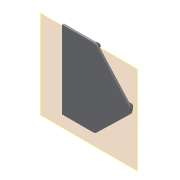
# Autodesk Inventor part: 20_Cube_Insert_VCM_MirrorMount_KES400A_mirror_mount
Saved by Autodesk Inventor 2019.4 (Build 234330000, 330)
## iProperties
Created: 2021-10-15
Part Number: 20_Cube_Insert_VCM_MirrorMount_KES400A_mirror_mount
Material: Generic
Document SubType Name: Modeling
Designer: diederichbenedict
Density: 1 g/cm^3
Appearance: Default
Author: diederichbenedict
Autodesk Inventor part; units mm, degrees
ref_plane "YZ Plane" through (0, 0, 0) normal (1, 0, 0) x (0, 1, 0)
ref_plane "XZ Plane" through (0, 0, 0) normal (0, 1, 0) x (-1, 0, 0)
ref_plane "XY Plane" through (0, 0, 0) normal (0, 0, 1) x (1, 0, 0)
ref_plane "Work Plane1" through (0, 0, -28) normal (0, 0, 1) x (1, 0, 0)
sketch "Sketch1" plane through (0, 0, -28) normal (0, 0, 1) x (1, 0, 0)
  circle A0 centre (27.88, 8) radius 2.6486 projected
  circle A1 centre (27.88, 43) radius 2.6486 projected
  circle A2 centre (44.7, 24.3248) radius 2.6486 projected
  line L0 (27.88, 8) -> (44.7, 24.3248)
  line L1 (44.7, 24.3248) -> (27.88, 43)
  line L2 (27.88, 43) -> (27.88, 8)
  line L3 (46.5446, 22.4242) -> (29.7246, 6.0994)
  line L4 (46.668, 26.0973) -> (29.848, 44.7725)
  line L5 (27.88, 5.3514) -> (11.88, 5.3514)
  line L6 (27.88, 5.3514) -> (43.88, 5.3514) construction
  line L7 (11.88, 5.3514) -> (11.88, 45.6486)
  line L8 (11.88, 45.6486) -> (27.88, 45.6486)
  point P0 (0, 0)
  dimension "d0" = 16
  dimension "d1" = 180
  constraints: 18 end point, 6 point on circle, 4 tangent, 3 perpendicular, 1 coincident, 1 collinear, 1 horizontal, 1 point on line, 1 vertical
  measures "d0" distance of L5.start L5.end
  measures "d1" angle of L5 L6
extrude "Extrusion1" add sketch "Sketch1" along normal blind 1
sketch "Sketch2" plane through (0, 0, -28) normal (0, 0, -1) x (-1, 0, 0)
  circle A0 centre (-44.7, 24.3248) radius 2.6486 projected
  circle A1 centre (-27.88, 43) radius 2.6486 projected
  circle A2 centre (-27.88, 8) radius 2.6486 projected
  point P0 (0, 0)
extrude "Extrusion2" add sketch "Sketch2" along normal blind 2 draft -40
body "Solid1"
